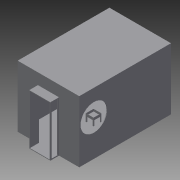
# Autodesk Inventor part: Bryant_Compartment
Saved by Autodesk Inventor 2013 SP2 (Build 170200200, 200)
## iProperties
Created: 2014-01-22
Part Number: Bryant_Compartment
Material: Generic
Document SubType Name: Modeling
Designer: mcgratta
Density: 1 g/cm^3
Author: mcgratta
Autodesk Inventor part; units mm, degrees
ref_plane "YZ Plane" through (0, 0, 0) normal (1, 0, 0) x (0, 1, 0)
ref_plane "XZ Plane" through (0, 0, 0) normal (0, 1, 0) x (-1, 0, 0)
ref_plane "XY Plane" through (0, 0, 0) normal (0, 0, 1) x (1, 0, 0)
sketch "Sketch1" plane through (0, 0, 0) normal (0, 1, 0) x (-1, 0, 0)
  line L0 (25, 25) -> (-3625, 25)
  line L1 (-3625, 25) -> (-3625, -2425)
  line L2 (-3625, -2425) -> (25, -2425)
  line L3 (25, -2425) -> (25, 25)
  point P0 (0, 0)
  dimension "d0" = 25
  dimension "d1" = 25
  dimension "d2" = 2450
  dimension "d3" = 3650
  constraints: 8 end point, 2 parallel, 1 horizontal, 1 perpendicular
  measures "d0" distance from line of point (0, 0) L3
  measures "d1" distance from line of point (0, 0) L0
  measures "d2" distance between parallel lines of L0 L2
  measures "d3" distance between parallel lines of L1 L3
extrude "Extrusion1" add sketch "Sketch1" along normal blind 25
sketch "Sketch2" plane through (0, 25, 0) normal (0, 1, 0) x (1, 0, 0)
  line L0 (3625, 2425) -> (-25, 2425) projected
  line L1 (-25, 2425) -> (-25, -25) projected
  line L2 (1645, 1355) -> (1675, 1355)
  line L3 (1675, 1355) -> (1675, 1385)
  line L4 (1675, 1385) -> (1645, 1385)
  line L5 (1645, 1385) -> (1645, 1355)
  line L6 (1925, 1355) -> (1955, 1355)
  line L7 (1955, 1355) -> (1955, 1385)
  line L8 (1955, 1385) -> (1925, 1385)
  line L9 (1925, 1385) -> (1925, 1355)
  line L10 (1925, 1075) -> (1955, 1075)
  line L11 (1955, 1075) -> (1955, 1105)
  line L12 (1955, 1105) -> (1925, 1105)
  line L13 (1925, 1105) -> (1925, 1075)
  line L14 (1645, 1075) -> (1675, 1075)
  line L15 (1675, 1075) -> (1675, 1105)
  line L16 (1675, 1105) -> (1645, 1105)
  line L17 (1645, 1105) -> (1645, 1075)
  point P0 (0, 0)
  dimension "d6" = 1670
  dimension "d7" = 1070
  dimension "d8" = 30
  dimension "d9" = 30
  dimension "d10" = 30
  dimension "d11" = 30
  dimension "d12" = 30
  dimension "d13" = 30
  dimension "d14" = 30
  dimension "d15" = 30
  dimension "d16" = 250
  dimension "d17" = 250
  dimension "d18" = 250
  dimension "d19" = 0
  dimension "d20" = 250
  dimension "d21" = 30
  constraints: 32 end point, 8 parallel, 4 horizontal, 4 perpendicular
  measures "d6" distance between parallel lines of L5 L1
  measures "d7" distance between parallel lines of L2 L0
  measures "d8" distance between parallel lines of L2 L4
  measures "d9" distance from line of L3.end L5
  measures "d10" distance between parallel lines of L6 L8
  measures "d11" distance from line of L7.end L9
  measures "d12" distance between parallel lines of L10 L12
  measures "d13" distance from line of L11.end L13
  measures "d14" distance between parallel lines of L14 L16
  measures "d15" distance from line of L15.end L17
  measures "d16" distance between parallel lines of L9 L3
  measures "d17" distance between parallel lines of L16 L2
  measures "d18" distance between parallel lines of L12 L6
  measures "d19" distance between parallel lines of L10 L14
  measures "d20" distance from line of L12.end L15
  measures "d21" distance between parallel lines of L8 L2
extrude "Extrusion2" add sketch "Sketch2" along normal blind 200
sketch "Sketch3" plane through (0, 225, 0) normal (0, 1, 0) x (1, 0, 0)
  line L0 (1645, 1385) -> (1955, 1385)
  line L1 (1955, 1385) -> (1955, 1075)
  line L2 (1955, 1075) -> (1645, 1075)
  line L3 (1645, 1075) -> (1645, 1385)
  point P0 (0, 0)
  dimension "d24" = 310
  dimension "d26" = 310
  constraints: 8 end point, 2 parallel, 1 horizontal, 1 perpendicular
  measures "d24" distance between parallel lines of L1 L3
  measures "d26" distance between parallel lines of L0 L2
extrude "Extrusion3" add sketch "Sketch3" along normal blind 100
sketch "Sketch4" plane through (0, 325, 0) normal (0, 1, 0) x (1, 0, 0)
  line L0 (1645, 1385) -> (1645, 1075) projected
  line L1 (1645, 1075) -> (1955, 1075) projected
  line L2 (1955, 1075) -> (1955, 1385) projected
  line L3 (1955, 1385) -> (1645, 1385) projected
  line L4 (1650, 1380) -> (1950, 1380)
  line L5 (1950, 1380) -> (1950, 1080)
  line L6 (1950, 1080) -> (1650, 1080)
  line L7 (1650, 1080) -> (1650, 1380)
  point P0 (0, 0)
  dimension "d29" = 5
  dimension "d30" = 5
  dimension "d31" = 5
  dimension "d32" = 5
  constraints: 8 end point, 2 parallel, 1 horizontal, 1 perpendicular
  measures "d29" distance between parallel lines of L7 L0
  measures "d30" distance between parallel lines of L3 L4
  measures "d31" distance between parallel lines of L2 L5
  measures "d32" distance between parallel lines of L1 L6
extrude "Extrusion4" cut sketch "Sketch4" against normal blind 90 contours L4 L5 L6 L7
sketch "Sketch5" plane through (0, 25, 0) normal (0, 1, 0) x (1, 0, 0)
  line L0 (-25, -25) -> (3625, -25) projected
  line L1 (3625, -25) -> (3625, 2425) projected
  line L2 (-25, -25) -> (3625, -25)
  line L3 (3625, -25) -> (3625, 2425)
  line L4 (3625, 2425) -> (-25, 2425)
  line L5 (-25, 2425) -> (-25, -25)
  line L6 (0, 0) -> (3600, 0)
  line L7 (3600, 0) -> (3600, 2400)
  line L8 (3600, 2400) -> (0, 2400)
  line L9 (0, 2400) -> (0, 0)
  dimension "d35" = 25
  dimension "d37" = 25
  constraints: 16 end point, 4 parallel, 2 horizontal, 2 perpendicular
  measures "d35" distance between parallel lines of L8 L4
  measures "d37" distance between parallel lines of L3 L7
extrude "Extrusion5" add sketch "Sketch5" along normal blind 2400
sketch "Sketch6" plane through (-25, 0, -2425) normal (-1, 0, 0) x (0, 0, 1)
  line L0 (0, 0) -> (2450, 0) projected
  line L1 (0, 0) -> (0, 2425) projected
  line L2 (830, 25) -> (1620, 25)
  line L3 (1620, 25) -> (1620, 1985)
  line L4 (1620, 1985) -> (830, 1985)
  line L5 (830, 1985) -> (830, 25)
  line L6 (805, 0) -> (1645, 0)
  line L7 (1645, 0) -> (1645, 2010)
  line L8 (1645, 2010) -> (805, 2010)
  line L9 (805, 2010) -> (805, 0)
  point P0 (2425, 0)
  dimension "d40" = 25
  dimension "d41" = 790
  dimension "d42" = 1960
  dimension "d43" = 830
  dimension "d44" = 25
  dimension "d45" = 25
  dimension "d46" = 25
  constraints: 16 end point, 4 parallel, 2 horizontal, 2 perpendicular, 1 point on line
  measures "d40" distance between parallel lines of L0 L2
  measures "d41" distance between parallel lines of L3 L5
  measures "d42" distance between parallel lines of L4 L2
  measures "d43" distance between parallel lines of L5 L1
  measures "d44" distance between parallel lines of L5 L9
  measures "d45" distance between parallel lines of L4 L8
  measures "d46" distance between parallel lines of L7 L3
extrude "Extrusion6" cut sketch "Sketch6" against normal blind 30 contours L5 L4 L3 L2
sketch "Sketch7" plane through (-25, 0, -2425) normal (-1, 0, 0) x (0, 0, 1)
  line L0 (1620, 1985) -> (1620, 25) projected
  line L1 (1620, 25) -> (830, 25) projected
  line L2 (830, 25) -> (830, 1985) projected
  line L3 (830, 1985) -> (1620, 1985) projected
  line L4 (0, 0) -> (2450, 0) projected
  line L5 (805, 0) -> (1645, 0)
  line L6 (1645, 0) -> (1645, 2010)
  line L7 (1645, 2010) -> (805, 2010)
  line L8 (805, 2010) -> (805, 0)
  point P0 (2425, 0)
  dimension "d49" = 25
  dimension "d50" = 25
  dimension "d51" = 25
  constraints: 8 end point, 2 parallel, 1 horizontal, 1 perpendicular, 1 point on line
  measures "d49" distance between parallel lines of L2 L8
  measures "d50" distance between parallel lines of L7 L3
  measures "d51" distance between parallel lines of L6 L0
extrude "Extrusion7" add sketch "Sketch7" along normal blind 345
sketch "Sketch8" plane through (-25, 0, 25) normal (0, 0, 1) x (1, 0, 0)
  circle A0 centre (580.5357, 1430.3643) radius 528.9159
  point P0 (25, 0)
  constraints: 1 centre point
extrude "Extrusion8" cut sketch "Sketch8" against normal blind 30
sketch "Sketch9" plane through (-25, 0, -780) normal (0, 0, 1) x (1, 0, 0)
  line L0 (0, 2010) -> (0, 0) projected
  line L1 (0, 2010) -> (-345, 2010) projected
  line L2 (-345, 0) -> (-345, 2010) projected
  line L3 (-295, 45) -> (-50, 45)
  line L4 (-50, 45) -> (-50, 1990)
  line L5 (-50, 1990) -> (-295, 1990)
  line L6 (-295, 1990) -> (-295, 45)
  line L7 (25, 25) -> (-345, 25) projected
  point P0 (25, 0)
  dimension "d56" = 50
  dimension "d57" = 20
  dimension "d58" = 20
  dimension "d59" = 50
  constraints: 8 end point, 2 parallel, 1 horizontal, 1 perpendicular
  measures "d56" distance between parallel lines of L2 L6
  measures "d57" distance between parallel lines of L1 L5
  measures "d58" distance between parallel lines of L7 L3
  measures "d59" distance between parallel lines of L0 L4
extrude "Extrusion9" cut sketch "Sketch9" against normal blind 30 contours L6 L5 L4 L3
sketch "Sketch10" plane through (-25, 0, 25) normal (0, 0, 1) x (1, 0, 0)
  line L0 (0, 2425) -> (3650, 2425)
  line L1 (3650, 2425) -> (3650, 2450)
  line L2 (3650, 2450) -> (0, 2450)
  line L3 (0, 2450) -> (0, 2425)
  point P0 (25, 0)
  dimension "d62" = 25
  dimension "d64" = 3650
  constraints: 8 end point, 2 parallel, 1 horizontal, 1 perpendicular
  measures "d62" distance between parallel lines of L0 L2
  measures "d64" distance of L1.end L2.end
extrude "Extrusion10" add sketch "Sketch10" against normal blind 2450
body "Solid1"
